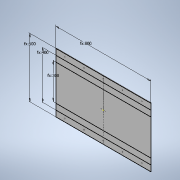
# Autodesk Inventor part: bolt_holes_for_all
Saved by Autodesk Inventor 2021 (Build 250183000, 183)
## iProperties
Created: 2021-02-10
Part Number: bolt_holes_for_all
Material: Generic
Document SubType Name: Modeling
Designer: pduy110
Density: 1 g/cm^3
Appearance: Default
Author: pduy110
Autodesk Inventor part; units mm, degrees
ref_plane "YZ Plane" through (0, 0, 0) normal (1, 0, 0) x (0, 1, 0)
ref_plane "XZ Plane" through (0, 0, 0) normal (0, 1, 0) x (-1, 0, 0)
ref_plane "XY Plane" through (0, 0, 0) normal (0, 0, 1) x (1, 0, 0)
sketch "base_layout_sketch" plane through (0, 0, 0) normal (0, 0, 1) x (1, 0, 0)
  line L0 (-400, 200) -> (400, 200)
  line L1 (400, 200) -> (400, -200)
  line L2 (400, -200) -> (-400, -200)
  line L3 (-400, -200) -> (-400, 200)
  line L4 (0, 200) -> (0, -200) construction
  line L5 (-400, 150) -> (400, 150)
  line L6 (400, 150) -> (400, -150)
  line L7 (400, -150) -> (-400, -150)
  line L8 (-400, -150) -> (-400, 150)
  line L9 (0, 150) -> (0, -150) construction
  line L10 (-400, 250) -> (400, 250)
  line L11 (400, 250) -> (400, -250)
  line L12 (400, -250) -> (-400, -250)
  line L13 (-400, -250) -> (-400, 250)
  line L14 (0, 250) -> (0, -250) construction
  point P0 (0, 0)
  point P1 (0, 0)
  dimension "d0" = 400
  dimension "d1" = 800
  dimension "d2" = 300
  dimension "d4" = 500
  constraints: 30 end point, 9 midpoint, 6 parallel, 3 horizontal, 3 perpendicular, 2 collinear, 1 coincident
  measures "d0" distance between parallel lines of L2 L0
  measures "d1" distance between parallel lines of L1 L3
  measures "d2" distance between parallel lines of L7 L5
  measures "d4" distance between parallel lines of L12 L10
sketch "bolt_holes_sketch" plane through (0, 0, 0) normal (0, 0, 1) x (1, 0, 0)
  circle A0 centre (-325, 225) radius 4
  line L0 (-400, 250) -> (400, 250) projected
  line L1 (-400, -250) -> (-400, 250) projected
  line L2 (-560, 0) -> (560, 0) projected
  point P0 (0, 0)
  dimension "d3" = 8
  dimension "d6" = 75
  dimension "d21" = 225
  constraints: 1 centre point
  measures "d3" diameter of A0
  measures "d6" distance from line of L1 A0.centre
  measures "d21" distance from line of L2 A0.centre
extrude "sheet_visualisation" add sketch "base_layout_sketch" against normal blind 5
extrude "bolt_holes Cut" cut sketch "bolt_holes_sketch" against normal through all
pattern_linear "bolt_holes_upper Pattern" count 5 spacing 162.5 along (1, 0, 0) of "bolt_holes Cut"
mirror "bolt_holes Mirror" about plane through (0, 0, 0) normal (0, 1, 0) of "bolt_holes Cut", "bolt_holes_upper Pattern"
equation "\"d0\" = layer_width"
equation "\"d1\" = track_length"
equation "\"d2\" = coil_width"
equation "\"d4\" = real_sheet_width"
equation "\"d3\" = bolt_diameter"
equation "\"d6\" = x_offset_for_bolts"
equation "\"d21\" = y_offset_for_bolts"
equation "\"d14\" = sheet_thickness"
equation "\"track_length\" = 800"
equation "\"layer_width\" = 400"
equation "\"coil_width\" = 300"
equation "\"bolt_diameter\" = 8"
equation "\"real_sheet_width\" = 500"
equation "\"x_offset_for_bolts\" = 75"
equation "\"y_offset_for_bolts\" = 225"
equation "\"sheet_thickness\" = 5"
body "Solid1"
